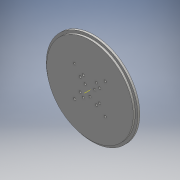
# Autodesk Inventor part: asztalv2
Saved by Autodesk Inventor 2016 (Build 200138000, 138)
## iProperties
Created: 2018-04-01
Part Number: asztalv2
Material: Generic
Document SubType Name: Modeling
Designer: bogna
Density: 1 g/cm^3
Appearance: Default
Author: bogna
Autodesk Inventor part; units mm, degrees
ref_plane "YZ Plane" through (0, 0, 0) normal (1, 0, 0) x (0, 1, 0)
ref_plane "XZ Plane" through (0, 0, 0) normal (0, 1, 0) x (-1, 0, 0)
ref_plane "XY Plane" through (0, 0, 0) normal (0, 0, 1) x (1, 0, 0)
sketch "Sketch1" plane through (0, 0, 0) normal (0, 0, 1) x (1, 0, 0)
  line L0 (0, -1.6) -> (0, 9.6) projected
  line L1 (-108, 0) -> (18, 0) projected
  line L2 (0, 0) -> (-85, 0)
  line L3 (-85, 0) -> (-85, 4)
  line L4 (-85, 4) -> (-90, 4)
  line L5 (-90, 4) -> (-90, 8)
  line L6 (0, 7.2) -> (0, 0)
  line L7 (-0.8, 8) -> (0, 7.2)
  line L8 (-18.8, 8) -> (-18, 7.2)
  line L9 (-18, 7.2) -> (-17.2, 8)
  line L10 (-90, 8) -> (-18.8, 8) construction
  line L11 (-17.2, 8) -> (-0.8, 8)
  line L12 (-36.8, 8) -> (-36, 7.2)
  line L13 (-36, 7.2) -> (-35.2, 8)
  line L14 (-54.8, 8) -> (-54, 7.2)
  line L15 (-54, 7.2) -> (-53.2, 8)
  line L16 (-72.8, 8) -> (-72, 7.2)
  line L17 (-72, 7.2) -> (-71.2, 8)
  line L18 (-18.8, 8) -> (-35.2, 8)
  line L19 (-36.8, 8) -> (-53.2, 8)
  line L20 (-54.8, 8) -> (-71.2, 8)
  line L21 (-72.8, 8) -> (-90, 8)
  point P0 (-18, 8)
  point P1 (-36, 8)
  point P2 (-54, 8)
  point P3 (-72, 8)
  dimension "d2" = 5
  dimension "d3" = 4
  dimension "d4" = 90
  dimension "d7" = 18
  dimension "d11" = 18
  dimension "d17" = 8
  dimension "d18" = 135
  dimension "d19" = 0.8
  constraints: 40 end point, 5 collinear, 4 perpendicular, 2 equal length, 2 parallel, 1 horizontal, 1 point on line, 1 vertical alignment, 18 other
  measures "d2" distance between parallel lines of L5 L3
  measures "d3" distance between parallel lines of L2 L4
  measures "d4" distance between parallel lines of L0 L5
  measures "d7" distance from line of L0 point (-18, 8)
  measures "d11" distance of L8.start L12.start
  measures "d17" distance between parallel lines of L2 L10
  measures "d18" angle of L7 L11
  measures "d19" distance from line of L11 L6.start
revolve "Revolution1" add sketch "Sketch1" angle 360 about axis through (0, -10, 0) along (0, 1, 0)
sketch "Sketch2" plane through (0, 8, 0) normal (0, 1, 0) x (1, 0, 0)
  line L0 (-30, 30) -> (30, 30) construction
  line L1 (30, 30) -> (30, -30) construction
  line L2 (30, -30) -> (-30, -30) construction
  line L3 (-30, -30) -> (-30, 30) construction
  line L4 (-19, 13) -> (19, 13) construction
  line L5 (19, 13) -> (19, -13) construction
  line L6 (19, -13) -> (-19, -13) construction
  line L7 (-19, -13) -> (-19, 13) construction
  line L8 (-13, 19) -> (13, 19) construction
  line L9 (13, 19) -> (13, -19) construction
  line L10 (13, -19) -> (-13, -19) construction
  line L11 (-13, -19) -> (-13, 19) construction
  line L12 (0, 126) -> (0, -126) projected
  line L13 (-126, 0) -> (126, 0) projected
  circle A0 centre (0, 0) radius 11 construction
  point P0 (0, 11)
  point P1 (-9.5263, -5.5)
  point P2 (9.5263, -5.5)
  dimension "d21" = 60
  dimension "d22" = 26
  dimension "d23" = 38
  dimension "d25" = 22
  dimension "d26" = 120
  dimension "d27" = 120
  constraints: 24 end point, 13 coincident, 6 parallel, 6 perpendicular, 3 horizontal, 3 point on circle, 2 midpoint, 1 centre point, 1 point on line, 6 other
  measures "d21" distance of L2.end L0.start
  measures "d22" distance of L8.start L8.end
  measures "d23" distance of L10.end L8.start
  measures "d25" diameter of A0
hole "Hole1" at (0, 8, -11) at (-9.5263, 8, 5.5) at (9.5263, 8, 5.5) at (-30, 8, -30) at (-19, 8, -13) at (-13, 8, -19) at (13, 8, -19) at (19, 8, -13) at (30, 8, -30) at (30, 8, 30) at (-30, 8, 30) at (-13, 8, 19) at (13, 8, 19) at (19, 8, 13) at (-19, 8, 13) direction (0, -1, 0) diameter 4.2 end through all
hole "Hole2" at (0, 8, -11) direction (0, -1, 0) diameter 4.2 end through all counterbore diameter 7.8 counterbore depth 3.2
pattern_circular "Circular Pattern1" count 3 over 360 about axis through (0, -10, 0) along (0, 1, 0) of "Hole2"
body "Solid1"
